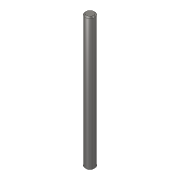
# Autodesk Inventor part: Arretierstift
Saved by Autodesk Inventor 2018.3 (Build 223284000, 284)
## iProperties
Created: 2019-11-28
Material: Stahl, Legierung
Document SubType Name: Modeling
Designer: dirkb
Density: 7.73 g/cm^3
Appearance: Halbpoliert
Description: Stift
Part Number: Arretierstift
Werkstoff: X8CrNiS18-9
Author: dirkb
Autodesk Inventor part; units mm, degrees
ref_plane "YZ Plane" through (0, 0, 0) normal (1, 0, 0) x (0, 1, 0)
ref_plane "XZ Plane" through (0, 0, 0) normal (0, 1, 0) x (-1, 0, 0)
ref_plane "XY Plane" through (0, 0, 0) normal (0, 0, 1) x (1, 0, 0)
sketch "Skizze_Grundkörper" plane through (0, 0, 0) normal (0, 0, 1) x (1, 0, 0)
  circle A0 centre (0, 0) radius 2
  dimension "d0" = 4
  constraints: 1 centre point, 1 coincident
  measures "d0" diameter of A0
extrude "Grudnkörper" add sketch "Skizze_Grundkörper" along normal mid plane 55
chamfer "Fase_0,5_mm" distance 0.5 angle 45 2 edges at (-2, 0, 27.5) (-2, 0, -27.5)
